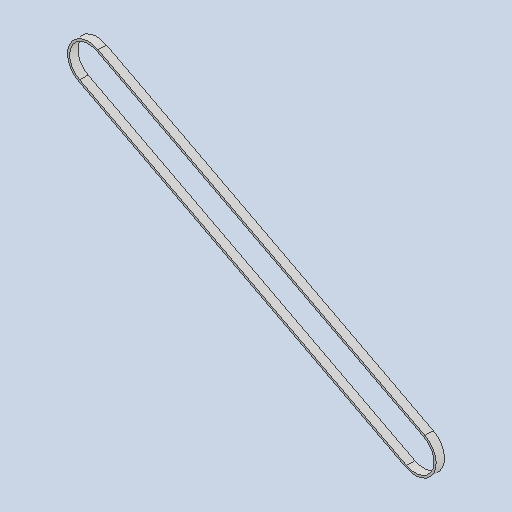
# Autodesk Inventor part: Lift up banding
Saved by Autodesk Inventor 2022.2 (Build 262287010, 287A)
## iProperties
Created: 2022-06-29
Part Number: Lift up banding
Material: Generic
Document SubType Name: Modeling
Designer: Main Account
Density: 1 g/cm^3
Appearance: Default
Author: Main Account
Autodesk Inventor part; units mm, degrees
ref_plane "YZ Plane" through (0, 0, 0) normal (1, 0, 0) x (0, 1, 0)
ref_plane "XZ Plane" through (0, 0, 0) normal (0, 1, 0) x (-1, 0, 0)
ref_plane "XY Plane" through (0, 0, 0) normal (0, 0, 1) x (1, 0, 0)
sketch "Sketch1" plane through (0, 0, 0) normal (0, 0, 1) x (1, 0, 0)
  circle A0 centre (-198.7719, 103.7404) radius 14.0335 construction
  arc A1 (-5.2885, -10.133) -> (5.2885, 10.133) centre (0, 0) ccw
  arc A2 (-5.8761, -11.2589) -> (5.8761, 11.2589) centre (0, 0) ccw
  arc A3 (-193.4834, 113.8734) -> (-204.0603, 93.6075) centre (-198.7719, 103.7404) ccw
  arc A4 (-192.8958, 114.9993) -> (-204.648, 92.4816) centre (-198.7719, 103.7404) ccw
  line L0 (-5.8761, -11.2589) -> (-204.648, 92.4816)
  line L1 (5.8761, 11.2589) -> (-192.8958, 114.9993)
  line L2 (-193.4834, 113.8734) -> (5.2885, 10.133)
  line L3 (-5.2885, -10.133) -> (-204.0603, 93.6075)
  dimension "d0" = 22.86
  dimension "d1" = 25.4
  dimension "d2" = 22.86
  dimension "d3" = 25.4
  constraints: 8 end point, 8 point on circle, 6 tangent, 4 centre point, 4 coincident, 2 parallel
  measures "d0" diameter of A1
  measures "d1" diameter of A2
  measures "d2" diameter of A3
  measures "d3" diameter of A4
extrude "Extrusion1" add sketch "Sketch1" against normal blind 5.08
body "Solid1"
